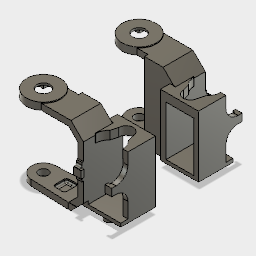
servo_bracket_knee_mirror (Autodesk Fusion 360 design; units mm, degrees)
Autodesk Fusion 360 part; units mm, degrees
note: some values were not read from the file. Set by a fixed rule: which sketch regions a step uses.
sketch "スケッチ1" plane through (0, 0, 0) normal (0, 1, 0) x (1, 0, 0)
  circle A0 centre (0, 0) radius 5.55
  circle A1 centre (0, 0) radius 2.75
  line L0 (2.75, 2.75) -> (-2.75, 2.75)
  line L1 (-2.75, 2.75) -> (-2.75, -2.75)
  line L2 (-2.75, -2.75) -> (2.75, -2.75)
  line L3 (2.75, -2.75) -> (2.75, 2.75)
  line L4 (2.75, 2.75) -> (-2.75, -2.75) construction
  line L5 (-2.75, 2.75) -> (2.75, -2.75) construction
  line L6 (-2.75, 2.75) -> (-4.8208, 2.75)
  line L7 (-2.75, -2.75) -> (-4.8208, -2.75)
  line L8 (-2.75, 2.75) -> (-2.75, 4.8208)
  line L9 (-2.75, -2.75) -> (-2.75, -4.8208)
  line L10 (2.75, -2.75) -> (4.8208, -2.75)
  line L11 (2.75, -2.75) -> (2.75, -4.8208)
  line L12 (2.75, 2.75) -> (4.8208, 2.75)
  line L13 (2.75, 2.75) -> (2.75, 4.8208)
  dimension "d1" = 11.1
  dimension "d2" = 5.5
  dimension "d3" = 5.5
  dimension "d4" = 5.5
  measures "d1" diameter of A0
  measures "d2" diameter of A1
  measures "d3" distance of L1.end L2.end
  measures "d4" distance of L0.end L1.end
sketch "スケッチ2" plane through (0, 0, 0) normal (0, 1, 0) x (1, 0, 0)
  circle A0 centre (0, 0) radius 7.15
  line L0 (5.5, 5.5) -> (-5.5, 5.5)
  line L1 (-5.5, 5.5) -> (-5.5, -5.5)
  line L2 (-5.5, -5.5) -> (5.5, -5.5)
  line L3 (5.5, -5.5) -> (5.5, 5.5)
  line L4 (5.5, 5.5) -> (-5.5, -5.5) construction
  line L5 (-5.5, 5.5) -> (5.5, -5.5) construction
  line L6 (0, 0) -> (22.2, 0)
  line L7 (5.5, -5.5) -> (5.5, 5.5)
  line L8 (5.5, 5.5) -> (22.2, 5.5)
  line L9 (22.2, 5.5) -> (22.2, -5.5)
  line L10 (22.2, -5.5) -> (5.5, -5.5)
  line L11 (22.2, -5.5) -> (19.88, -5.5)
  line L12 (19.88, -5.5) -> (19.88, 5.5)
  line L13 (19.88, 5.5) -> (22.2, 5.5)
  line L14 (22.2, 5.5) -> (22.2, -5.5)
  dimension "d5" = 14.3
  dimension "d6" = 11
  dimension "d7" = 11
  dimension "d8" = 22.2
  dimension "d9" = 2.32
  measures "d5" diameter of A0
  measures "d6" distance of L0.end L1.end
  measures "d7" distance of L1.end L2.end
  measures "d8" distance of A0.centre L6.end
  measures "d9" distance of L9.end L11.end
extrude "押し出し1" add sketch "スケッチ2" against normal blind 3 contours A0 L3 L6 L7 | A0 L3 L6 L7 | A0 L0 L1 L2 L3 L7 | A0 L0 | A0 L2 | A0 L1 makes body 1
extrude "押し出し2" cut sketch "スケッチ1" against normal blind 5.5 contours A0 L3 L10 L12 | A0 L0 L8 L13 | A1 L0 L3 | A0 L2 L9 L11 | A1 L2 L3 | A1 | A1 L0 L1 | A1 L1 L2 | A0 L1 L6 L7 bodies 1
extrude "押し出し3" add sketch "スケッチ1" against normal blind 0.8 contours A0 L3 L10 L12 | A0 L0 L8 L13 | A1 L0 L3 | A0 L2 L9 L11 | A1 L2 L3 | A1 L0 L1 | A1 L1 L2 | A0 L1 L6 L7 bodies 1
extrude "押し出し4" add sketch "スケッチ2" against normal blind 3 contours A0 L3 L6 L7 L10 L12 | A0 L3 L6 L7 L8 L12 | A0 L0 L3 L7 | A0 L2 L3 L7 bodies 1
extrude "押し出し5" add sketch "スケッチ2" against normal blind 33.1 contours L6 L8 L9 L12 L13 L14 | L6 L9 L10 L11 L12 L14 bodies 1
extrude "押し出し6" cut sketch "スケッチ2" against normal blind 0.4 contours A0 L3 L6 L7 L10 L12 | A0 L3 L6 L7 L8 L12 | A0 L0 L3 L7 | A0 L2 L3 L7 | L6 L8 L9 L12 L13 L14 | L6 L9 L10 L11 L12 L14 bodies 1
ref_plane "作業平面1" through (0, -32.7, 0) normal (0, 1, 0) x (1, 0, 0)
sketch "スケッチ3" plane through (0, -33.1, 0) normal (0, -1, 0) x (1, 0, 0)
  circle A0 centre (0, 0) radius 2
  circle A1 centre (0, 0) radius 5
  line L0 (0, 0) -> (16, 0)
  line L1 (16, -5.6065) -> (-0.1883, -4.9965)
  line L2 (19.88, 5.5) -> (19.88, -5.6065)
  line L3 (19.88, -5.6065) -> (16, -5.6065)
  line L4 (16, -5.6065) -> (16, 0)
  line L5 (19.88, 5.5) -> (9.2, 5.5)
  line L6 (19.88, 5.5) -> (30.56, 5.5) construction
  line L7 (9.2, 5.5) -> (-0.2675, 4.9928)
  line L8 (19.88, -5.5) -> (22.2, -5.5)
  line L9 (22.2, -5.5) -> (22.2, 5.5)
  line L10 (22.2, 5.5) -> (19.88, 5.5)
  line L11 (19.88, 5.5) -> (19.88, -5.5)
  point P0 (19.88, 5.5)
  point P1 (19.88, -5.5)
  dimension "d23" = 4
  dimension "d24" = 10
  dimension "d25" = 16
  dimension "d26" = 180
  dimension "d27" = 10.68
  dimension "d121" = 3.88
  measures "d23" diameter of A0
  measures "d24" diameter of A1
  measures "d25" distance of A0.centre L0.end
  measures "d26" angle of L5 L6
  measures "d27" distance of L5.end P0
  measures "d121" distance of L2.end L1.start
extrude "押し出し7" add sketch "スケッチ3" along normal blind -2.6 and the other way blind 0 contours A1 | A1 L0 L1 L4 | A1 L0 L2 L3 L4 L5 L7 L11 bodies 1
sketch "スケッチ4" plane through (0, 0, 0) normal (0, 1, 0) x (1, 0, 0)
  line L0 (22.2, -5.5) -> (22.2, -7)
  line L1 (22.2, -5.5) -> (23.7, -5.5) construction
  line L2 (22.2, -7) -> (9.2, -7)
  line L3 (22.2, -7) -> (35.2, -7) construction
  line L4 (9.2, -7) -> (9.2, -5.5)
  line L5 (22.2, -5.5) -> (9.2, -5.5)
  point P0 (9.2, -5.5)
  point P1 (22.2, -5.5)
  point P2 (22.2, -5.5)
  point P3 (9.2, -5.5)
  point P4 (9.2, -5.5)
  dimension "d32" = 90
  dimension "d33" = 1.5
  dimension "d34" = 180
  dimension "d35" = 13
  measures "d32" angle of L0 L1
  measures "d33" distance of L0.start L0.end
  measures "d34" angle of L2 L3
  measures "d35" distance of L0.end L2.end
extrude "押し出し9" add sketch "スケッチ4" against normal blind 33.1 bodies 1
extrude "押し出し10" cut sketch "スケッチ4" against normal blind 0.4 bodies 1
chamfer "面取り1" distance 3.88 angle 45 2 edges at (19.88, -3, 0) (19.88, -30.5, 0) on bodies 1
chamfer "面取り2" distance 5.2 angle 45 2 edges at (22.2, -0.4, 0.75) (22.2, -33.1, 0.75) on bodies 1
ref_plane "作業平面2" through (22.2, -16.55, 0.75) normal (1, 0, 0) x (0, 0, 1)
sketch "スケッチ5" plane through (22.2, -16.55, 0.75) normal (1, 0, 0) x (0, 0, -1)
  line L0 (6.25, -13.95) -> (-4.75, -13.95)
  line L1 (5.7465, -13.95) -> (-4.2428, -13.95)
  line L2 (-6.25, -11.35) -> (-6.25, -16.55)
  line L3 (-2.7394, -13.95) -> (-11.2658, -13.95)
sketch "スケッチ6" plane through (22.2, -16.55, 0.75) normal (1, 0, 0) x (0, 0, -1)
  line L0 (-6.25, -11.35) -> (-6.25, -16.55)
  line L1 (-6.25, -13.95) -> (-6.25, -14.15)
  line L2 (-6.25, -13.95) -> (-6.05, -13.95) construction
  line L3 (-6.25, -14.15) -> (-10.25, -14.15)
  line L4 (-6.25, -14.15) -> (-2.25, -14.15) construction
  line L5 (-10.25, -14.15) -> (-6.25, -14.15)
  line L6 (-6.25, -14.15) -> (-6.25, 11.65)
  line L7 (-6.25, 11.65) -> (-10.25, 11.65)
  line L8 (-10.25, 11.65) -> (-10.25, -14.15)
  line L9 (-6.25, -14.15) -> (4.25, -14.15)
  line L10 (4.25, -14.15) -> (4.25, -12.65)
  line L11 (4.25, -12.65) -> (-6.25, -12.65)
  line L12 (-6.25, -12.65) -> (-6.25, -14.15)
  line L13 (-6.25, 11.65) -> (1.25, 11.65)
  line L14 (1.25, 11.65) -> (1.25, 8.15)
  line L15 (1.25, 8.15) -> (-6.25, 8.15)
  line L16 (-6.25, 8.15) -> (-6.25, 11.65)
  line L17 (-6.25, 8.15) -> (-10.25, 8.15)
  line L18 (-6.25, -12.65) -> (-10.25, -12.65)
  dimension "d43" = 90
  dimension "d45" = 180
  dimension "d46" = 4
  dimension "d47" = 25.8
  dimension "d48" = 10.5
  dimension "d49" = 1.5
  dimension "d50" = 7.5
  dimension "d51" = 3.5
  measures "d43" angle of L1 L2
  measures "d45" angle of L3 L4
  measures "d46" distance of L1.end L3.end
  measures "d47" distance of L3.end L7.end
  measures "d48" distance of L1.end L9.end
  measures "d49" distance of L1.end L11.end
  measures "d50" distance of L6.end L13.end
  measures "d51" distance of L6.end L15.end
extrude "押し出し11" add sketch "スケッチ6" along normal blind 2.32 separate body contours L0 L6 L8 L17 L18 makes body 2
extrude "押し出し12" add sketch "スケッチ6" along normal blind 15.92 contours L0 L1 L6 L9 L10 L11 L12 | L0 L1 L3 L5 L6 L8 L12 L18 | L6 L7 L8 L16 L17 | L6 L13 L14 L15 L16 bodies 2
extrude "押し出し13" cut sketch "スケッチ6" along normal blind 2.32 contours L0 L1 L6 L9 L10 L11 L12 | L6 L13 L14 L15 L16 bodies 2
sketch "スケッチ7" plane through (38.12, 0, 0) normal (1, 0, 0) x (0, 0, -1)
  line L0 (0.5, -4.9) -> (-11, -4.9)
  line L1 (-11, -4.9) -> (-11, -8.4)
  line L2 (-11, -8.4) -> (0.5, -8.4)
  line L3 (0.5, -8.4) -> (0.5, -4.9)
  line L4 (-11, -4.9) -> (0.5, -4.9)
  line L5 (0.5, -4.9) -> (0.5, -30.7)
  line L6 (0.5, -30.7) -> (-11, -30.7)
  line L7 (-11, -30.7) -> (-11, -4.9)
  point P0 (-11, -4.9)
  dimension "d58" = 11.5
  dimension "d59" = 25.8
  measures "d58" distance of P0 L0.start
  measures "d59" distance of P0 L6.end
extrude "押し出し14" add sketch "スケッチ7" against normal blind 2 contours L2 L5 L6 L7 bodies 2
sketch "スケッチ8" plane through (0, -4.9, 0) normal (0, 1, 0) x (-1, 0, 0)
  line L0 (-24.52, 7) -> (-22.2, 7)
  line L1 (-22.2, 7) -> (-22.2, 11)
  line L2 (-22.2, 11) -> (-38.12, 11)
  line L3 (-38.12, 11) -> (-38.12, -0.5)
  line L4 (-38.12, -0.5) -> (-24.52, -0.5)
  line L5 (-24.52, -0.5) -> (-24.52, 7)
  line L6 (-24.52, -0.5) -> (-30.32, -0.5)
  line L7 (-24.52, -0.5) -> (-18.72, -0.5) construction
  circle A0 centre (-30.32, -0.5) radius 5.6
  line L8 (-30.32, -0.5) -> (-30.32, 6.5)
  line L9 (-30.32, -0.5) -> (-37.32, -0.5) construction
  circle A1 centre (-30.32, 6.5) radius 3
  line L10 (-30.32, 6.5) -> (-27.32, 6.5)
  line L11 (-30.32, 6.5) -> (-33.32, 6.5)
  line L12 (-27.32, 6.5) -> (-26.5193, 3.6127)
  line L13 (-27.32, 6.5) -> (-24.3238, 6.5) construction
  line L14 (-33.32, 6.5) -> (-34.1207, 3.6127)
  dimension "d62" = 180
  dimension "d63" = 5.8
  dimension "d64" = 11.2
  dimension "d65" = 90
  dimension "d66" = 7
  dimension "d67" = 6
  dimension "d68" = 74.5
  dimension "d69" = 105.5
  measures "d62" angle of L6 L7
  measures "d63" distance of L4.end L6.end
  measures "d64" diameter of A0
  measures "d65" angle of L8 L9
  measures "d66" distance of L6.end L8.end
  measures "d67" diameter of A1
  measures "d68" angle of L12 L13
  measures "d69" angle of L13 L14
extrude "押し出し15" cut sketch "スケッチ8" against normal blind 7.5 contours L4 L6 A0 L8 A1 | L4 A0 L8 A1 | A0 A1 L12 | A0 L8 A1 | A0 L8 A1 | A0 L8 A1 L10 | A1 L10 L11 | A0 A1 L14 | A0 L8 A1 L11 bodies 2
sketch "スケッチ9" plane through (0, -30.7, 0) normal (0, -1, 0) x (1, 0, 0)
  line L0 (38.12, -3.5) -> (38.12, 11)
  line L1 (38.12, 11) -> (22.2, 11)
  line L2 (22.2, 11) -> (22.2, 7)
  line L3 (22.2, 7) -> (24.52, 7)
  line L4 (24.52, 7) -> (24.52, -3.5)
  line L5 (24.52, -3.5) -> (38.12, -3.5)
  circle A0 centre (30.32, -0.5) radius 1.9
  point P0 (30.32, -0.5)
  dimension "d72" = 3.8
  measures "d72" diameter of A0
extrude "押し出し16" add sketch "スケッチ9" along normal blind 2.4 contours A0 bodies 2
sketch "スケッチ10" plane through (36.12, 0, 0) normal (-1, 0, 0) x (0, 0, 1)
  line L0 (-0.5, -29.2) -> (11, -29.2)
  line L1 (11, -29.2) -> (11, -8.4)
  line L2 (11, -8.4) -> (-0.5, -8.4)
  line L3 (-0.5, -8.4) -> (-0.5, -29.2)
  line L4 (-0.5, -4.9) -> (-0.5, -14.7)
  line L5 (-0.5, -4.9) -> (9.3, -4.9) construction
  line L6 (-0.5, -14.7) -> (-7.3, -14.7)
  line L7 (-7.3, -14.7) -> (-7.3, -17.8)
  line L8 (-7.3, -17.8) -> (-0.5, -17.8)
  line L9 (-0.5, -17.8) -> (-0.5, -14.7)
  line L10 (-7.3, -17.8) -> (-6.1, -17.8)
  line L11 (-6.1, -17.8) -> (-6.1, -14.7)
  line L12 (-6.1, -14.7) -> (-7.3, -14.7)
  line L13 (-7.3, -14.7) -> (-7.3, -17.8)
  point P0 (-0.5, -4.9)
  dimension "d75" = 90
  dimension "d76" = 9.8
  dimension "d77" = 3.1
  dimension "d79" = 1.2
  dimension "d97" = 5.6
  measures "d75" angle of L4 L5
  measures "d76" distance of P0 L4.end
  measures "d77" distance of L4.end L8.end
  measures "d79" distance of L7.end L10.end
  measures "d97" distance of L9 L11
extrude "押し出し17" add sketch "スケッチ10" against normal blind 2 contours L3 L6 L8 L9 L11 | L6 L7 L8 L10 L11 L12 L13 bodies 2
extrude "押し出し18" add sketch "スケッチ10" along normal blind 0.8 contours L6 L7 L8 L10 L11 L12 L13 bodies 2
sketch "スケッチ11" plane through (19.88, 0, 0) normal (-1, 0, 0) x (0, 0, 1)
  line L0 (5.5, -26.62) -> (5.5, -6.88)
  line L1 (5.5, -6.88) -> (-5.5, -6.88)
  line L2 (-5.5, -6.88) -> (-5.5, -26.62)
  line L3 (-7.3, -17.8) -> (-6.1, -17.8)
  line L4 (-6.1, -17.8) -> (-6.1, -14.7)
  line L5 (-6.1, -14.7) -> (-7.5, -14.7)
  line L6 (-7.3, -14.7) -> (-7.3, -17.8)
  line L7 (-0.5, -14.7) -> (-7.3, -14.7)
  line L8 (-5.5, -14.7) -> (-5.5, -12.7)
  line L9 (-5.5, -14.7) -> (-7.5, -14.7) construction
  line L10 (-5.5, -12.7) -> (-6.1, -12.7)
  line L11 (-6.1, -12.7) -> (-6.1, -19.8)
  line L12 (-6.1, -19.8) -> (-5.5, -19.8)
  line L13 (-5.5, -19.8) -> (-5.5, -12.7)
  line L14 (-7.3, -14.7) -> (-7.3, -17.8)
  line L15 (-7.3, -17.8) -> (-7.3, -14.7)
  line L16 (-5.5, -26.62) -> (5.5, -26.62)
  point P0 (-7.3, -17.8)
  point P1 (-6.1, -14.7)
  dimension "d84" = 90
  dimension "d85" = 2
  dimension "d86" = 7.1
  dimension "d87" = 0.6
  measures "d84" angle of L8 L9
  measures "d85" distance of L8.start L8.end
  measures "d86" distance of L8.end L12.end
  measures "d87" distance of L8.end L10.end
extrude "押し出し19" add sketch "スケッチ11" against normal blind 2.32 contours L2 L4 L7 L11 L12 L13 | L2 L7 L8 L10 L11 L13 | L3 L4 L5 L6 L7 L11 L14 L15 bodies 1
extrude "押し出し20" add sketch "スケッチ11" against normal blind 3.12 contours L3 L4 L5 L6 L7 L11 L14 L15 bodies 1
move_body "ボディを移動1" bodies 2 to x (1, 0, 0) y (0, 1, 0) z (0, 0, 1) at (-2.32, 0, 0)
combine "結合1" operation add target body 1 tool bodies 2
sketch "スケッチ12" plane through (0, -30.7, 0) normal (0, -1, 0) x (1, 0, 0)
  circle A0 centre (28, -0.5) radius 1.9
  line L0 (35.8, -3.5) -> (35.8, 11)
  line L1 (35.8, 11) -> (19.88, 11)
  line L2 (19.88, 11) -> (19.88, 7)
  line L3 (19.477, -3.5) -> (19.477, 7)
  line L4 (19.477, 7) -> (22.2, 7)
  line L5 (19.88, 7) -> (22.2, 7)
  line L6 (22.2, 7) -> (22.2, -3.5)
  line L7 (19.477, -3.5) -> (22.2, -3.5)
  line L8 (22.2, 7) -> (22.2, -3.5)
  point P0 (22.2, 7)
  point P1 (22.2, -3.5)
  dimension "d94" = 2.723
  measures "d94" distance of P0 L3.end
extrude "押し出し21" add sketch "スケッチ12" against normal blind 3.5 contours L3 L4 L5 L6 L7 L8 bodies 1
ref_plane "作業平面3" through (27.84, -17.8, 20) normal (0, 0, 1) x (0, -1, 0)
fillet "フィレット1" radius 5 2 edges at (34.8, -17.8, -0.5) (34.8, -14.7, -0.5) on bodies 1
fillet "フィレット2" radius 1 2 edges at (21.04, -17.8, -6.1) (21.04, -14.7, -6.1) on bodies 1
sketch "スケッチ13" plane through (0, -30.5, 0) normal (0, 1, 0) x (-1, 0, 0)
  line L0 (-16, -5.6065) -> (0.1883, -4.9965)
  arc A0 (0.1883, -4.9965) -> (0.2675, 4.9928) centre (0, 0) ccw
  line L1 (0.2675, 4.9928) -> (-9.2, 5.5)
  line L2 (-11.7, -2.9427) -> (-6.7, -2.7543)
  line L3 (-6.7, -2.7543) -> (-6.7, 2.8661)
  line L4 (-11.7, 3) -> (-11.7, -2.9427)
  line L5 (-6.7, 2.8661) -> (-9.2, 3)
  line L6 (-9.2, 3) -> (-11.7, 3)
  circle A1 centre (0, 0) radius 2
  line L7 (-19.6, -5.5) -> (-19.6, -5.6065)
  line L8 (-19.6, -5.6065) -> (-16, -5.6065)
  line L9 (-16, -5.5) -> (-19.6, -5.5)
  dimension "d119" = 2.5
  dimension "d122" = 2.5
  dimension "d123" = 2.5
  dimension "d124" = 2.5
  measures "d119" distance of L0 L2
  measures "d122" distance of L1.end L4
  measures "d123" distance of L1.end L3
  measures "d124" distance of L1.end L5.end
extrude "押し出し22" cut sketch "スケッチ13" against normal blind 1.5 contours L2 L3 L4 L5 L6 bodies 1
sketch "スケッチ14" plane through (0, -3, 0) normal (0, -1, 0) x (1, 0, 0)
  line L0 (9.2, 5.5) -> (4.5686, 5.5)
  arc A0 (4.5686, 5.5) -> (4.5686, -5.5) centre (0, 0) ccw
  line L1 (4.5686, -5.5) -> (16, -5.5)
  arc A1 (4.8208, -2.75) -> (4.8208, 2.75) centre (0, 0) ccw
  line L2 (4.8208, -2.75) -> (2.75, -2.75)
  line L3 (2.75, -2.75) -> (2.75, -4.8208)
  arc A2 (-2.75, -4.8208) -> (2.75, -4.8208) centre (0, 0) ccw
  line L4 (-2.75, -4.8208) -> (-2.75, -2.75)
  line L5 (-2.75, -2.75) -> (-4.8208, -2.75)
  arc A3 (-4.8208, 2.75) -> (-4.8208, -2.75) centre (0, 0) ccw
  line L6 (-4.8208, 2.75) -> (-2.75, 2.75)
  line L7 (-2.75, 2.75) -> (-2.75, 4.8208)
  arc A4 (2.75, 4.8208) -> (-2.75, 4.8208) centre (0, 0) ccw
  line L8 (2.75, 4.8208) -> (2.75, 2.75)
  line L9 (2.75, 2.75) -> (4.8208, 2.75)
  line L10 (6.7, 3) -> (11.7, 3)
  line L11 (11.7, 3) -> (11.7, -3)
  line L12 (11.7, -3) -> (6.7, -3)
  line L13 (6.7, -3) -> (6.7, 3)
  line L14 (16, -5.5) -> (16, 5.5)
  line L15 (16, 5.5) -> (9.2, 5.5)
  dimension "d107" = 2.5
  dimension "d109" = 2.5
  dimension "d110" = 5
  measures "d107" distance of L1 L12
  measures "d109" distance of L0.start L13
  measures "d110" distance of L10.start L10.end
extrude "押し出し23" cut sketch "スケッチ14" against normal blind 1.5 contours L10 L11 L12 L13 bodies 1
fillet "フィレット3" radius 1 17 edges at (11.7, -2.25, 3) (6.7, -2.25, 3) (11.7, -2.25, -3) (9.2, -1.5, -3) (11.7, -1.5, 0) (6.7, -2.25, -3) (6.7, -1.5, 0) (9.2, -1.5, 3) (10.45, -32, 3) (7.95, -32, 2.933) (11.7, -31.25, 3) (11.7, -32, 0.0287) (9.2, -32, -2.8485) (11.7, -31.25, -2.9427) (6.7, -32, 0.0559) (6.7, -31.25, -2.7543) (6.7, -31.25, 2.8661) on bodies 1
mirror "ミラー2" about plane through (27.84, -17.8, 20) normal (0, 0, 1) of bodies 1 makes body 3
sketch "スケッチ15" plane through (19.477, 0, 0) normal (-1, 0, 0) x (0, 0, 1)
  line L0 (-3.5, -30.623) -> (-3.5, -30.7)
  line L1 (7, -30.623) -> (-3.5, -30.623)
  line L2 (-3.5, -30.7) -> (7, -30.7)
  line L3 (7, -30.7) -> (7, -30.623)
equation "d82 = 1 mm - 0.2 mm"
equation "d90 = -3.32 mm + 0.2 mm"
named bodies: "ボディ2"
